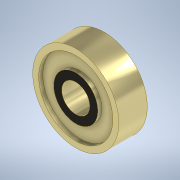
# Autodesk Inventor part: Cojinete
Saved by Autodesk Inventor 2022 (Build 260153000, 153)
## iProperties
Created: 2022-01-31
Part Number: Cojinete
Material: Generic
Document SubType Name: Modeling
Designer: hurta
Density: 1 g/cm^3
Appearance: Gold - Metal
Author: hurta
Autodesk Inventor part; units mm, degrees
ref_plane "YZ Plane" through (0, 0, 0) normal (1, 0, 0) x (0, 1, 0)
ref_plane "XZ Plane" through (0, 0, 0) normal (0, 1, 0) x (-1, 0, 0)
ref_plane "XY Plane" through (0, 0, 0) normal (0, 0, 1) x (1, 0, 0)
sketch "Sketch1" plane through (0, 0, 0) normal (0, 0, 1) x (1, 0, 0)
  circle A0 centre (0, 0) radius 3.5
  circle A1 centre (0, 0) radius 10.75
  dimension "d0" = 7
  dimension "d1" = 21.5
  constraints: 2 centre point, 2 coincident
  measures "d0" diameter of A0
  measures "d1" diameter of A1
extrude "Extrusion1" add sketch "Sketch1" along normal blind 5.1
sketch "Sketch2" plane through (0, 0, 5.1) normal (0, 0, 1) x (1, 0, 0)
  circle A0 centre (0, 0) radius 10.75 projected
  circle A1 centre (0, 0) radius 3.5 projected
  circle A2 centre (0, 0) radius 5.5
  circle A3 centre (0, 0) radius 9.25
  dimension "d4" = 11
  dimension "d5" = 18.5
  constraints: 2 centre point, 2 coincident
  measures "d4" diameter of A2
  measures "d5" diameter of A3
sketch "Sketch3" plane through (0, 0, 0) normal (0, 0, -1) x (-1, 0, 0)
  circle A0 centre (0, 0) radius 9.25 projected
  circle A1 centre (0, 0) radius 5.5 projected
  circle A2 centre (0, 0) radius 3.5 projected
  circle A3 centre (0, 0) radius 10.75 projected
extrude "Extrusion2" add sketch "Sketch3" along normal blind 1
extrude "Extrusion3" add sketch "Sketch2" along normal blind 1
body "Solid1"
